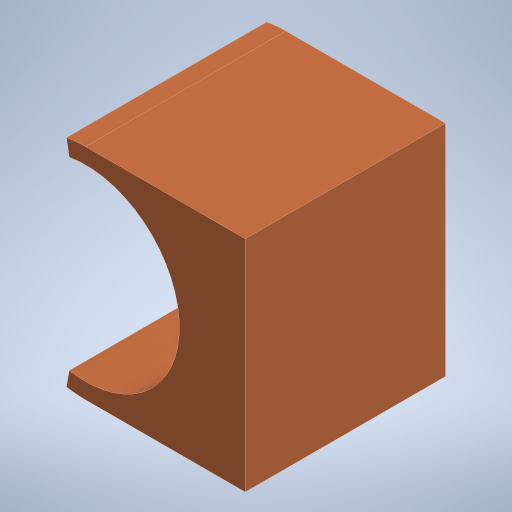
# Autodesk Inventor part: hook-thingy-base
Saved by Autodesk Inventor 2023.1 (Build 271208000, 208)
## iProperties
Created: 2023-03-31
Part Number: hook-thingy-base
Material: Generic
Document SubType Name: Modeling
Designer: caleb
Density: 1 g/cm^3
Appearance: Default
Author: caleb
Autodesk Inventor part; units mm, degrees
ref_plane "YZ Plane" through (0, 0, 0) normal (1, 0, 0) x (0, 1, 0)
ref_plane "XZ Plane" through (0, 0, 0) normal (0, 1, 0) x (-1, 0, 0)
ref_plane "XY Plane" through (0, 0, 0) normal (0, 0, 1) x (1, 0, 0)
sketch "Sketch1" plane through (0, 0, 0) normal (0, 0, 1) x (1, 0, 0)
  line L0 (-2.0675, -11.7254) -> (-2.4148, -13.695)
  arc A0 (-2.4148, -13.695) -> (-2.4148, 13.695) centre (0, 0) ccw
  line L1 (-2.4148, 13.695) -> (-2.0675, 11.7254)
  arc A1 (-2.0675, -11.7254) -> (-2.0675, 11.7254) centre (0, 0) ccw
  line L2 (0, 13.9062) -> (20.2562, 13.9062)
  line L3 (20.2562, 13.9062) -> (20.2562, -13.9062)
  line L4 (20.2562, -13.9062) -> (0, -13.9062)
  line L5 (13.9062, 13.9062) -> (13.9063, -13.9062) construction
  line L6 (17.0812, 13.9062) -> (17.0813, -13.9062) construction
  dimension "d0" = 11.9062
  dimension "d1" = 2
  dimension "d2" = 160
  dimension "d3" = 6.35
  dimension "d4" = 3.175
  constraints: 14 end point, 6 point on circle, 6 point on line, 4 perpendicular, 3 tangent, 2 centre point, 2 vertical alignment, 1 coincident, 1 concentric, 1 horizontal
  measures "d0" radius of A1
  measures "d1" distance of L1.start L1.end
  measures "d2" angle of L0 L1
  measures "d3" distance between parallel lines of L3 L5
  measures "d4" distance between parallel lines of L3 L6
extrude "Extrusion1" add sketch "Sketch1" along normal blind 25.4
ref_plane "mirror-plane" through (17.0812, 13.9062, 0) normal (1, 0, 0) x (0, 0, -1)
equation "\"d4\" = 0.5 * d3"
